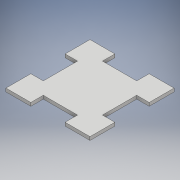
# Autodesk Inventor part: Pokrywka
Saved by Autodesk Inventor 2018 (Build 220112000, 112)
## iProperties
Created: 2018-10-19
Part Number: Pokrywka
Material: Ogólny
Document SubType Name: Modeling
Designer: EWA
Density: 1 g/cm^3
Appearance: Domyślna
Author: EWA
Autodesk Inventor part; units mm, degrees
ref_plane "YZ Plane" through (0, 0, 0) normal (1, 0, 0) x (0, 1, 0)
ref_plane "XZ Plane" through (0, 0, 0) normal (0, 1, 0) x (-1, 0, 0)
ref_plane "XY Plane" through (0, 0, 0) normal (0, 0, 1) x (1, 0, 0)
sketch "Szkic1" plane through (0, 0, 0) normal (0, 0, 1) x (1, 0, 0)
  line L0 (0, 0) -> (152, 0) construction
  line L1 (152, 0) -> (152, 152) construction
  line L2 (152, 152) -> (0, 152) construction
  line L3 (0, 152) -> (0, 0) construction
  line L4 (129.5, 22.5) -> (22.5, 22.5) construction
  line L5 (22.5, 22.5) -> (22.5, 129.5) construction
  line L6 (22.5, 129.5) -> (129.5, 129.5) construction
  line L7 (129.5, 129.5) -> (129.5, 22.5) construction
  line L8 (0, 0) -> (45, 0) construction
  line L9 (45, 0) -> (45, 45) construction
  line L10 (45, 45) -> (0, 45) construction
  line L11 (0, 45) -> (0, 0) construction
  line L12 (0, 152) -> (45, 152) construction
  line L13 (45, 152) -> (45, 107) construction
  line L14 (45, 107) -> (0, 107) construction
  line L15 (0, 107) -> (0, 152) construction
  line L16 (152, 152) -> (107, 152) construction
  line L17 (107, 152) -> (107, 107) construction
  line L18 (107, 107) -> (152, 107) construction
  line L19 (152, 107) -> (152, 152) construction
  line L20 (152, 0) -> (107, 0) construction
  line L21 (107, 0) -> (107, 45) construction
  line L22 (107, 45) -> (152, 45) construction
  line L23 (152, 45) -> (152, 0) construction
  line L24 (0, 0) -> (45, 0)
  line L25 (45, 0) -> (45, 22.5)
  line L26 (45, 22.5) -> (107, 22.5)
  line L27 (107, 22.5) -> (107, 0)
  line L28 (107, 0) -> (152, 0)
  line L29 (152, 0) -> (152, 45)
  line L30 (152, 45) -> (129.5, 45)
  line L31 (129.5, 45) -> (129.5, 107)
  line L32 (129.5, 107) -> (152, 107)
  line L33 (152, 107) -> (152, 152)
  line L34 (152, 152) -> (107, 152)
  line L35 (107, 152) -> (107, 129.5)
  line L36 (107, 129.5) -> (45, 129.5)
  line L37 (45, 129.5) -> (45, 152)
  line L38 (45, 152) -> (0, 152)
  line L39 (0, 152) -> (0, 107)
  line L40 (0, 107) -> (22.5, 107)
  line L41 (22.5, 107) -> (22.5, 45)
  line L42 (22.5, 45) -> (0, 45)
  line L43 (0, 45) -> (0, 0)
  dimension "d0" = 152
  dimension "d1" = 152
  dimension "d2" = 22.5
  dimension "d3" = 45
  dimension "d4" = 45
  dimension "d5" = 45
  dimension "d6" = 45
  dimension "d7" = 45
  dimension "d8" = 45
  dimension "d9" = 45
  dimension "d10" = 45
  constraints: 88 end point, 12 parallel, 11 perpendicular, 8 midpoint, 7 collinear, 5 horizontal, 3 other
  measures "d0" distance of L2.end L1.end
  measures "d1" distance of L1.end L0.end
  measures "d2" distance between parallel lines of L0 L4
  measures "d3" distance of L10.end L9.end
  measures "d4" distance of L9.end L8.end
  measures "d5" distance of L12.end L13.end
  measures "d6" distance of L17.end L16.end
  measures "d7" distance of L17.end L18.end
  measures "d8" distance of L13.end L14.end
  measures "d9" distance of L21.end L22.end
  measures "d10" distance of L20.end L21.end
extrude "Wyciągnięcie proste1" add sketch "Szkic1" along normal blind 6
equation "\"d1\" = d0"
